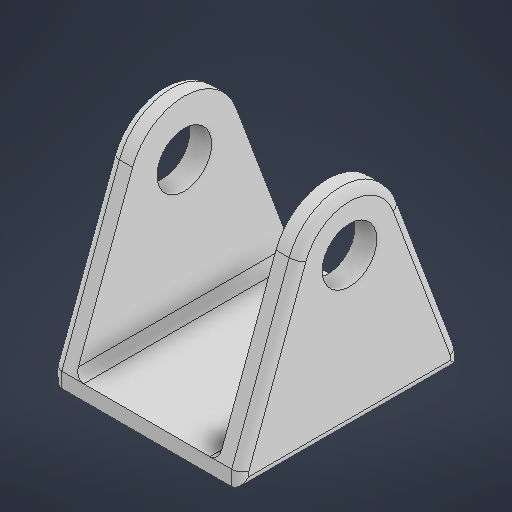
# Autodesk Inventor part: largebracket
Saved by Autodesk Inventor 2026.2 (Build 302298010, 298A)
## iProperties
Created: 2026-08-01
Part Number: largebracket
Material: Generic
Document SubType Name: Modeling
Designer: tasle
Density: 1 g/cm^3
Appearance: Default
Author: tasle
Autodesk Inventor part; units mm, degrees
ref_plane "YZ Plane" through (0, 0, 0) normal (1, 0, 0) x (0, 1, 0)
ref_plane "XZ Plane" through (0, 0, 0) normal (0, 1, 0) x (-1, 0, 0)
ref_plane "XY Plane" through (0, 0, 0) normal (0, 0, 1) x (1, 0, 0)
sketch "Sketch1" plane through (0, 0, 0) normal (1, 0, 0) x (0, 1, 0)
  circle A0 centre (0, 0) radius 6.35
  line L0 (0, 0) -> (-34.925, 0)
  line L1 (-34.925, 25.4) -> (-34.925, -25.4)
  line L2 (-34.925, 25.4) -> (-31.425, 25.4)
  line L3 (-31.425, 25.4) -> (-31.425, -25.4)
  line L4 (-31.425, -25.4) -> (-34.925, -25.4)
  line L5 (-34.925, -25.4) -> (-34.925, 25.4)
  circle A1 centre (0, 0) radius 12.827
  line L6 (4.4793, 12.0195) -> (-31.425, 25.4)
  line L7 (4.4793, -12.0195) -> (-31.425, -25.4)
  dimension "d0" = 12.7
  dimension "d1" = 34.925
  dimension "d2" = 50.8
  dimension "d3" = 3.5
  dimension "d4" = 25.654
  constraints: 16 end point, 2 centre point, 2 coincident, 2 horizontal, 2 parallel, 2 point on circle, 2 tangent, 1 midpoint, 1 perpendicular, 1 vertical
  measures "d0" diameter of A0
  measures "d1" distance of L0.start L0.end
  measures "d2" distance of L1.start L1.end
  measures "d3" distance of L3.end L4.end
  measures "d4" diameter of A1
extrude "Extrusion1" add sketch "Sketch1" along normal blind 43.4975 contours L3 L4 L1 L0 | L0 L1 L2 L3
sketch "Sketch2" plane through (43.4975, 0, 0) normal (1, 0, 0) x (0, 0, -1)
  line L0 (-25.4, -34.925) -> (25.4, -34.925) projected
  line L1 (25.4, -34.925) -> (25.4, -31.425) projected
  line L2 (25.4, -31.425) -> (-25.4, -31.425) projected
  line L3 (-25.4, -31.425) -> (-25.4, -34.925) projected
  line L4 (-25.4, -31.425) -> (-25.4, -34.925) projected
  line L5 (-25.4, -34.925) -> (25.4, -34.925) projected
  line L6 (-25.4, -31.425) -> (-25.4, -34.925) projected
  line L7 (25.4, -31.425) -> (-25.4, -31.425) projected
  line L8 (25.4, -34.925) -> (25.4, -31.425) projected
  line L9 (-25.4, -31.425) -> (-25.4, -34.925) projected
  line L10 (-25.4, -31.425) -> (-25.4, -34.925) projected
  circle A0 centre (0, 0) radius 6.35 projected
  line L11 (0, 0) -> (0, -34.925) projected
  line L12 (-25.4, -34.925) -> (25.4, -34.925) projected
  line L13 (-25.4, -34.925) -> (-25.4, -31.425) projected
  line L14 (-25.4, -31.425) -> (25.4, -31.425) projected
  line L15 (25.4, -31.425) -> (25.4, -34.925) projected
  line L16 (25.4, -34.925) -> (-25.4, -34.925) projected
  circle A1 centre (0, 0) radius 12.827 projected
  line L17 (-12.0195, 4.4793) -> (-25.4, -31.425) projected
  line L18 (12.0195, 4.4793) -> (25.4, -31.425) projected
  constraints: 3 other
extrude "Extrusion2" add sketch "Sketch1" along normal blind 5.08 contours A1 | A1 L7 L3 L0 | L0 L3 L6 A1
extrude "Extrusion3" add sketch "Sketch2" against normal blind 5.08 contours L17 A1 L11 L2 | L11 A1 L18 L2 | A1
fillet "Fillet1" radius 2 14 edges at (43.4975, 12.827, 0) (43.4975, -13.4728, -18.7097) (43.4975, -13.4728, 18.7097) (0, 12.827, 0) (0, -13.4728, -18.7097) (0, -13.4728, 18.7097) (43.4975, -33.175, 25.4) (43.4975, -33.175, -25.4) (0, -33.175, 25.4) (0, -33.175, -25.4) (43.4975, -34.925, 0) (0, -34.925, 0) (38.4175, -31.425, 0) (5.08, -31.425, 0)
body "Solid1"
